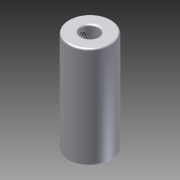
# Autodesk Inventor part: Roller
Saved by Autodesk Inventor 2012 (Build 160160000, 160)
## iProperties
Created: 2012-10-03
Part Number: Roller
Material: Default
Document SubType Name: Modeling
Designer: agmlego
Density: 1 g/cm^3
Author: agmlego
Autodesk Inventor part; units mm, degrees
ref_plane "XZ Plane" through (0, 0, 0) normal (0, 1, 0) x (-1, 0, 0)
ref_plane "XY Plane" through (0, 0, 0) normal (0, 0, 1) x (1, 0, 0)
sketch "Sketch1" plane through (0, 0, 0) normal (0, 0, 1) x (1, 0, 0)
  circle A0 centre (0, 0) radius 6.35
  dimension "d0" = 12.7
  constraints: 1 centre point, 1 coincident
  measures "d0" diameter of A0
extrude "Extrusion1" add sketch "Sketch1" along normal blind 30
hole "Hole1" at (0, 0, 30) direction (0, 0, -1) diameter 5 depth 10 tip angle 118
fillet "Fillet1" radius 0.5 3 edges at (0, 2.5, 30) (-6.35, 0, 30) (-6.35, 0, 0)
ref_plane "Work Plane1" through (-6.35, 0, 0) normal (1, 0, 0) x (0, 1, 0)
sketch "Sketch2" plane through (-6.35, 0, 0) normal (1, 0, 0) x (0, 1, 0)
  line L0 (0, 50.0021) -> (0, 0) construction
  line L1 (-5.85, 30) -> (5.85, 30) construction
  point P0 (0, 27.5)
  point P1 (0, 22.5)
  dimension "d23" = 2.5
  dimension "d24" = 5
  constraints: 2 end point, 2 point on line, 1 vertical
  measures "d23" distance from line of L1 point (0, 27.5)
  measures "d24" distance of point (0, 27.5) point (0, 22.5)
hole "Hole3" at (-6.35, 0, 27.5) at (-6.35, 0, 22.5) direction (1, 0, 0) diameter 2.156 end up to face face through (0, 0, 25) facing (0, 0, 1) round with radius 2.5 far side no thread size "4-40 UNC" class "2B" standard "ANSI Unified Screw Threads"
fillet "Fillet2" radius 0.5 4 edges at (-6.2578, 1.078, 27.4975) (-6.2578, -1.078, 27.4972) (-6.2578, -1.078, 22.4972) (-6.2578, 1.078, 22.4975)
body "Solid1"
